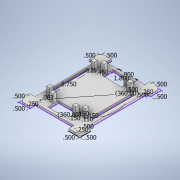
# Autodesk Inventor part: PixfalconCover
Saved by Autodesk Inventor 2020 (Build 240168000, 168)
## iProperties
Created: 2019-06-13
Part Number: PixfalconCover
Material: Generic
Document SubType Name: Sheet Metal
Designer: amirt
Density: 1 g/cm^3
Sheet Metal Rule: Default
Appearance: Default
Author: amirt
Autodesk Inventor part; units mm, degrees
ref_plane "YZ Plane" through (0, 0, 0) normal (1, 0, 0) x (0, 1, 0)
ref_plane "XZ Plane" through (0, 0, 0) normal (0, 1, 0) x (-1, 0, 0)
ref_plane "XY Plane" through (0, 0, 0) normal (0, 0, 1) x (1, 0, 0)
sketch "Sketch1" plane through (0, 0, 0) normal (0, 1, 0) x (-1, 0, 0)
  line L0 (45.72, 0) -> (45.72, -69.85)
  line L1 (0, -69.85) -> (0, 0)
  line L2 (45.72, -69.85) -> (58.42, -69.85)
  line L3 (58.42, -69.85) -> (58.42, -82.55)
  line L4 (58.42, -82.55) -> (45.72, -82.55)
  line L5 (45.72, -82.55) -> (45.72, -69.85)
  line L6 (45.72, 0) -> (58.42, 0)
  line L7 (58.42, 0) -> (58.42, 12.7)
  line L8 (58.42, 12.7) -> (45.72, 12.7)
  line L9 (45.72, 12.7) -> (45.72, 0)
  line L10 (0, 0) -> (-12.7, 0)
  line L11 (-12.7, 0) -> (-12.7, 12.7)
  line L12 (-12.7, 12.7) -> (0, 12.7)
  line L13 (0, 12.7) -> (0, 0)
  line L14 (0, -69.85) -> (-12.7, -69.85)
  line L15 (-12.7, -69.85) -> (-12.7, -82.55)
  line L16 (-12.7, -82.55) -> (0, -82.55)
  line L17 (0, -82.55) -> (0, -69.85)
  line L18 (0, 0) -> (0, 6.35)
  line L19 (0, 6.35) -> (45.72, 6.35)
  line L20 (45.72, 6.35) -> (45.72, 0)
  line L21 (0, -69.85) -> (0, -76.2)
  line L22 (0, -76.2) -> (45.72, -76.2)
  line L23 (45.72, -76.2) -> (45.72, -69.85)
  line L24 (45.72, -69.85) -> (52.07, -69.85)
  line L25 (52.07, -69.85) -> (52.07, 0)
  line L26 (52.07, 0) -> (45.72, 0)
  line L27 (45.72, 0) -> (45.72, -69.85)
  line L28 (0, 0) -> (-8.636, 0)
  line L29 (-8.636, 0) -> (-8.636, -69.85)
  line L30 (-8.636, -69.85) -> (0, -69.85)
  line L31 (0, -69.85) -> (0, 0)
  line L32 (0, 3.175) -> (0, -9.525)
  line L33 (45.72, -9.525) -> (45.72, 3.175)
  line L34 (0, -73.025) -> (0, -60.325)
  line L35 (45.72, -60.325) -> (45.72, -73.025)
  line L36 (34.29, -60.325) -> (11.43, -60.325)
  line L37 (11.43, -60.325) -> (11.43, -73.025)
  line L38 (11.43, -73.025) -> (34.29, -73.025)
  line L39 (34.29, -73.025) -> (34.29, -60.325)
  line L40 (34.29, -9.525) -> (11.43, -9.525)
  line L41 (11.43, -9.525) -> (11.43, 3.175)
  line L42 (11.43, 3.175) -> (34.29, 3.175)
  line L43 (34.29, 3.175) -> (34.29, -9.525)
  line L44 (11.43, -3.175) -> (7.62, -3.175)
  line L45 (7.62, -3.175) -> (7.62, -6.985)
  line L46 (7.62, -6.985) -> (11.43, -6.985)
  line L47 (11.43, -6.985) -> (11.43, -3.175)
  line L48 (0, -6.985) -> (3.81, -6.985)
  line L49 (3.81, -6.985) -> (3.81, -10.795)
  line L50 (3.81, -10.795) -> (0, -10.795)
  line L51 (0, -10.795) -> (0, -6.985)
  line L52 (38.1, -62.865) -> (34.29, -62.865)
  line L53 (38.1, -66.675) -> (38.1, -62.865)
  line L54 (34.29, -66.675) -> (38.1, -66.675)
  line L55 (45.72, -62.865) -> (41.91, -62.865)
  line L56 (41.91, -62.865) -> (41.91, -59.055)
  line L57 (41.91, -59.055) -> (45.72, -59.055)
  line L58 (7.62, -62.865) -> (11.43, -62.865)
  line L59 (7.62, -66.675) -> (7.62, -62.865)
  line L60 (11.43, -66.675) -> (7.62, -66.675)
  line L61 (0, -62.865) -> (3.81, -62.865)
  line L62 (3.81, -62.865) -> (3.81, -59.055)
  line L63 (3.81, -59.055) -> (0, -59.055)
  line L64 (41.91, -10.795) -> (45.72, -10.795)
  line L65 (41.91, -6.985) -> (41.91, -10.795)
  line L66 (45.72, -6.985) -> (41.91, -6.985)
  line L67 (38.1, -6.985) -> (34.29, -6.985)
  line L68 (38.1, -3.175) -> (38.1, -6.985)
  line L69 (34.29, -3.175) -> (38.1, -3.175)
  line L70 (36.195, -10.795) -> (9.525, -10.795)
  line L71 (9.525, -10.795) -> (9.525, -59.055)
  line L72 (9.525, -59.055) -> (36.195, -59.055)
  line L73 (36.195, -59.055) -> (36.195, -10.795)
  line L74 (47.3075, -10.795) -> (50.4825, -10.795)
  line L75 (50.4825, -10.795) -> (50.4825, -59.055)
  line L76 (50.4825, -59.055) -> (47.3075, -59.055)
  line L77 (47.3075, -59.055) -> (47.3075, -10.795)
  line L78 (22.86, -34.925) -> (22.86, -41.845)
  line L79 (-1.5875, -10.795) -> (-4.7625, -10.795)
  line L80 (-4.7625, -10.795) -> (-4.7625, -59.055)
  line L81 (-4.7625, -59.055) -> (-1.5875, -59.055)
  line L82 (-1.5875, -59.055) -> (-1.5875, -10.795)
  dimension "d0" = 45.72
  dimension "d1" = 69.85
  dimension "d2" = 12.7
  dimension "d3" = 12.7
  dimension "d4" = 12.7
  dimension "d5" = 12.7
  dimension "d6" = 12.7
  dimension "d7" = 12.7
  dimension "d8" = 12.7
  dimension "d9" = 12.7
  dimension "d10" = 6.35
  dimension "d11" = 6.35
  dimension "d12" = 6.35
  dimension "d13" = 12.7
  dimension "d14" = 12.7
  dimension "d15" = 11.43
  dimension "d16" = 22.86
  dimension "d17" = 12.7
  dimension "d18" = 3.81
  dimension "d19" = 3.81
  dimension "d20" = 3.81
  dimension "d21" = 3.81
  dimension "d24" = 360
  dimension "d28" = 360
  dimension "d34" = 1.5875
  dimension "d35" = 3.175
  constraints: 166 end point, 27 parallel, 11 horizontal, 11 perpendicular, 8 point on line, 6 midpoint, 4 symmetric about line, 1 vertical, 58 other
  measures "d0" distance of L0.end L1.start
  measures "d1" distance of L0.start L0.end
  measures "d2" distance of L3.end L4.end
  measures "d3" distance of L2.end L3.end
  measures "d4" distance of L8.end L7.end
  measures "d5" distance of L7.end L6.end
  measures "d6" distance of L11.end L12.end
  measures "d7" distance of L10.end L11.end
  measures "d8" distance of L16.end L15.end
  measures "d9" distance of L15.end L14.end
  measures "d10" distance of L18.start L18.end
  measures "d11" distance of L21.end L21.start
  measures "d12" distance of L26.end L25.end
  measures "d13" distance of L32.end L32.start
  measures "d14" distance of L34.start L34.end
  measures "d15" distance of L35.start L36.start
  measures "d16" distance of L38.end L37.end
  measures "d17" distance of L37.end L36.end
  measures "d18" distance of L46.end L45.end
  measures "d19" distance of L45.end L44.end
  measures "d20" distance of L49.end L50.end
  measures "d21" distance of L48.end L49.end
  measures "d34" distance of L64.end L74.start
  measures "d35" distance of L75.end L76.end
extrude "Extrusion1" add sketch "Sketch1" along normal blind 2.54 contours L6 L25 L2 L0 | L9 L8 L7 L6 | L0 L66 L65 L64 L57 L56 L55 L5 L22 L17 L1 L61 L62 L63 L50 L49 L48 L13 L19 L9 | L2 L3 L4 L5 | L13 L10 L11 L12 | L1 L14 L29 L10 | L17 L16 L15 L14 | L73 L72 L71 L70
extrude "Extrusion2" add sketch "Sketch1" along normal blind 12.7 contours L0 L64 L65 L66 | L0 L55 L56 L57 | L48 L49 L50 L1 | L1 L63 L62 L61 | L52 L53 L54 L39 | L37 L60 L59 L58 | L43 L69 L68 L67 | L46 L45 L44 L41
fillet "Fillet1" radius 6.35 4 edges at (-58.42, 1.27, 12.7) (12.7, 1.27, 12.7) (12.7, 1.27, -82.55) (-58.42, 1.27, -82.55)
equation "\"BendRadius\" = Thickness"
equation "\"BendReliefWidth\" = Thickness"
equation "\"BendReliefDepth\" = 0.5 * Thickness"
equation "\"CornerReliefSize\" = 4 * Thickness"
equation "\"MinimumRemnant\" = 2 * Thickness"
equation "\"TransitionRadius\" = BendRadius"
equation "\"JacobiRadiusSize\" = BendRadius"
equation "\"GapSize\" = Thickness"
equation "\"Thickness\" = 3.048"
body "Solid1"
